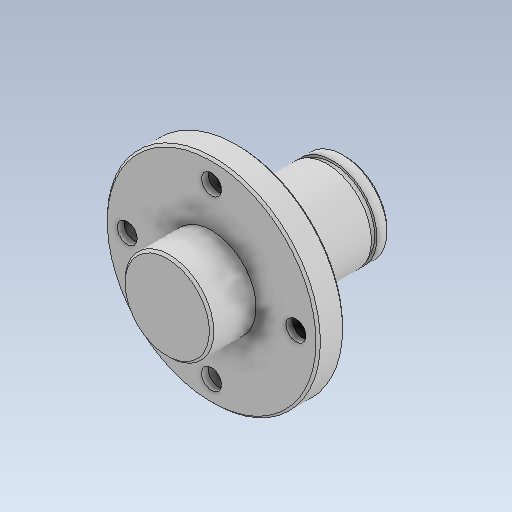
# Autodesk Inventor part: Peça41
Saved by Autodesk Inventor 2021 (Build 250183000, 183)
## iProperties
Category: 41
Created: 2021-07-23
Part Number: Peça41
Material: Genérico
Document SubType Name: Modeling
Designer: Giovanni
Density: 1 g/cm^3
Appearance: Padrão
User Status: 1:1
Author: Giovanni
Keywords: 24
Autodesk Inventor part; units mm, degrees
ref_plane "YZ Plane" through (0, 0, 0) normal (1, 0, 0) x (0, 1, 0)
ref_plane "XZ Plane" through (0, 0, 0) normal (0, 1, 0) x (-1, 0, 0)
ref_plane "XY Plane" through (0, 0, 0) normal (0, 0, 1) x (1, 0, 0)
sketch "Esboço1" plane through (0, 0, 0) normal (0, 0, 1) x (1, 0, 0)
  circle A0 centre (0, 0) radius 24
  dimension "d0" = 48
  constraints: 1 centre point, 1 coincident
  measures "d0" diameter of A0
extrude "Extrusão1" add sketch "Esboço1" along normal blind 6
sketch "Esboço2" plane through (0, 0, 6) normal (0, 0, 1) x (1, 0, 0)
  circle A0 centre (0, 0) radius 24 projected
  circle A1 centre (0, 0) radius 10
  dimension "d3" = 20
  constraints: 1 centre point, 1 coincident
  measures "d3" diameter of A1
extrude "Extrusão2" add sketch "Esboço2" along normal blind 10 contours A1
sketch "Esboço3" plane through (0, 0, 0) normal (0, 0, -1) x (-1, 0, 0)
  circle A0 centre (0, 0) radius 24 projected
  circle A1 centre (0, 0) radius 14
  dimension "d6" = 28
  constraints: 1 centre point, 1 coincident
  measures "d6" diameter of A1
extrude "Extrusão3" add sketch "Esboço3" along normal blind 4 contours A1
sketch "Esboço4" plane through (0, 0, -4) normal (0, 0, -1) x (-1, 0, 0)
  circle A0 centre (0, 0) radius 14 projected
  circle A1 centre (0, 0) radius 10
  dimension "d9" = 20
  constraints: 1 centre point, 1 coincident
  measures "d9" diameter of A1
extrude "Extrusão4" add sketch "Esboço4" along normal blind 20 contours A1
sketch "Esboço5" plane through (0, 0, 0) normal (1, 0, 0) x (0, 1, 0)
  line L0 (10, -20) -> (9.5, -20)
  line L1 (9.5, -20) -> (9.5, -21.25)
  line L2 (9.5, -21.25) -> (10, -21.25)
  line L3 (10, -21.25) -> (10, -20)
  line L4 (-10, -24) -> (10, -24) projected
  line L5 (0, -32) -> (0, 24) projected
  point P0 (0, 0)
  dimension "d12" = 1.25
  dimension "d13" = 4
  dimension "d14" = 9.5
  constraints: 8 end point, 2 parallel, 1 horizontal, 1 perpendicular, 1 vertical alignment
  measures "d12" distance between parallel lines of L2 L0
  measures "d13" distance between parallel lines of L0 L4
  measures "d14" horizontal distance of point (0, 0) L0.end
revolve "Revolução1" cut sketch "Esboço5" angle 360 about axis through (0, 0, -10) along (0, 0, 1)
sketch "Esboço6" plane through (0, 0, 0) normal (0, 0, -1) x (-1, 0, 0)
  circle A0 centre (0, 0) radius 14 projected
  point P0 (19, 0)
  dimension "d16" = 19
  constraints: 1 horizontal alignment
  measures "d16" distance of A0.centre point (19, 0)
hole "Furo1" at (-19, 0, 0) direction (0, 0, 1) diameter 4.5 end through all counterbore diameter 8 counterbore depth 4.5 clearance for "Socket Head Cap Screw DIN EN ISO 4762" size "M4" standard "DIN"
pattern_circular "Padrão circular1" count 4 over 360 about axis through (0, 0, 0) along (0, 0, 1) of "Furo1"
chamfer "Chanfro1" distance 0.5 angle 45 5 edges at (-10, 0, 16) (-24, 0, 6) (-24, 0, 0) (14, 0, -4) (10, 0, -24)
